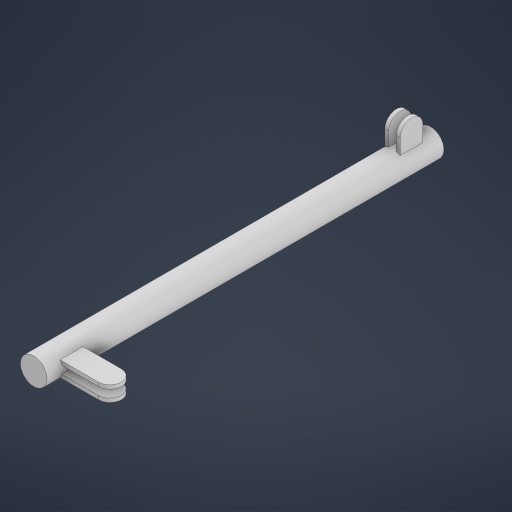
# Autodesk Inventor part: driveshaft_m_mount
Saved by Autodesk Inventor 2023 (Build 270158000, 158)
## iProperties
Created: 2023-09-20
Part Number: driveshaft_m_mount
Material: Generic
Document SubType Name: Modeling
Designer: Peter
Density: 1 g/cm^3
Appearance: Default
Author: Peter
Autodesk Inventor part; units mm, degrees
ref_plane "YZ Plane" through (0, 0, 0) normal (1, 0, 0) x (0, 1, 0)
ref_plane "XZ Plane" through (0, 0, 0) normal (0, 1, 0) x (-1, 0, 0)
ref_plane "XY Plane" through (0, 0, 0) normal (0, 0, 1) x (1, 0, 0)
sketch "Sketch1" plane through (0, 0, 0) normal (0, 0, 1) x (1, 0, 0)
  circle A0 centre (0, 0) radius 44.45
  dimension "d0" = 88.9
  constraints: 1 centre point, 1 coincident
  measures "d0" diameter of A0
extrude "Extrusion1" add sketch "Sketch1" along normal blind 1320.8
sketch "Sketch2" plane through (0, 0, 0) normal (0, 1, 0) x (-1, 0, 0)
  line L0 (12.7, 50.8) -> (25.4, 50.8)
  line L1 (25.4, 50.8) -> (25.4, 127)
  line L2 (25.4, 127) -> (12.7, 127)
  line L3 (12.7, 127) -> (12.7, 50.8)
  line L4 (0, -25.4) -> (0, 152.4) construction
  line L5 (-12.7, 50.8) -> (-25.4, 50.8)
  line L6 (-25.4, 50.8) -> (-25.4, 127)
  line L7 (-25.4, 127) -> (-12.7, 127)
  line L8 (-12.7, 127) -> (-12.7, 50.8)
  point P0 (0, 0)
  dimension "d3" = 76.2
  dimension "d4" = 12.7
  dimension "d5" = 12.7
  dimension "d6" = 50.8
  constraints: 16 end point, 4 symmetric about line, 2 parallel, 1 horizontal, 1 perpendicular
  measures "d3" distance of L0.end L1.end
  measures "d4" distance of L1.end L2.end
  measures "d5" distance between parallel lines of L4 L3
  measures "d6" distance from line of point (0, 0) L0
extrude "Extrusion2" add sketch "Sketch2" along normal blind 127
sketch "Sketch3" plane through (0, 0, 0) normal (1, 0, 0) x (0, 1, 0)
  line L0 (12.7, 1270) -> (25.4, 1270)
  line L1 (25.4, 1270) -> (25.4, 1193.8)
  line L2 (25.4, 1193.8) -> (12.7, 1193.8)
  line L3 (12.7, 1193.8) -> (12.7, 1270)
  line L4 (0, -264.16) -> (0, 1584.96) construction
  line L5 (44.45, 1320.8) -> (-44.45, 1320.8) construction
  line L6 (-12.7, 1270) -> (-25.4, 1270)
  line L7 (-25.4, 1270) -> (-25.4, 1193.8)
  line L8 (-25.4, 1193.8) -> (-12.7, 1193.8)
  line L9 (-12.7, 1193.8) -> (-12.7, 1270)
  point P0 (0, 0)
  point P1 (19.05, 1270)
  point P2 (-19.05, 1270)
  dimension "d10" = 12.7
  dimension "d11" = 12.7
  dimension "d12" = 76.2
  dimension "d13" = 50.8
  constraints: 16 end point, 5 symmetric about line, 2 parallel, 1 horizontal, 1 midpoint, 1 perpendicular
  measures "d10" distance between parallel lines of L4 L3
  measures "d11" distance of L0.start L0.end
  measures "d12" distance of L0.end L1.end
  measures "d13" distance from line of L5 point (19.05, 1270)
extrude "Extrusion3" add sketch "Sketch3" along normal blind 203.2
fillet "Fillet1" radius 38.1 8 edges at (-19.05, 127, 127) (19.05, 127, 127) (19.05, 127, 50.8) (-19.05, 127, 50.8) (203.2, 19.05, 1270) (203.2, 19.05, 1193.8) (203.2, -19.05, 1193.8) (203.2, -19.05, 1270)
body "Solid1"
